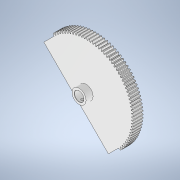
# Autodesk Inventor part: Spur Gear2
Saved by Autodesk Inventor 2020 (Build 240168000, 168)
## iProperties
CustomPartVersion: 1
Created: 2020-05-17
Part Number: Spur Gear2
Material: Acetal Resin, White
Document SubType Name: Modeling
Designer: Hesekiel
Categories: <?xml version="1.0" encoding="UTF-16"?> <MemberInstance><Categories><FamilyTemplate><FamilyTemplateParameter ValueType="xs:double" Id="1" ObjectReferenceKey="da_z" ObjectType="kUserParameterObject"/><FamilyTemplateParameter ValueType="xs:double" Id="2" ObjectReferenceKey="da_b" ObjectType="kUserParameterObject"/><FamilyTemplateParameter ValueType="xs:double" Id="3" ObjectReferenceKey="da_beta" ObjectType="kUserParameterObject"/><FamilyTemplateParameter ValueType="xs:double" Id="4" ObjectReferenceKey="da_da" ObjectType="kUserParameterObject"/><FamilyTemplateParameter ValueType="xs:double" Id="5" ObjectReferenceKey="da_aw" ObjectType="kUserParameterObject"/><FamilyTemplateParameter ValueType="xs:string" Id="6" ObjectReferenceKey="EAIAABAAAACIAQAAAAAAAIAAAAAAAAAA" ObjectType="83910656" SubObjectId="SurfaceGeometry"/></FamilyTemplate><ParamToTemplateMap><ParamToTemplate CategoryParameter="//CategoryParameter[@InternalName='046C89C9-8512-4d59-83FE-43B91F4F132A']" TemplateParameter="1"/><ParamToTemplate CategoryParameter="//CategoryParameter[@InternalName='2552DF32-E462-4b46-AEBF-C6C7768E72AC']" TemplateParameter="2"/><ParamToTemplate CategoryParameter="//CategoryParameter[@InternalName='C9EE641D-15FC-4fae-A226-E94C4372FDD7']" TemplateParameter="3"/><ParamToTemplate><ParamToTemplate CategoryParameter="//CategoryParameter[@InternalName='00B6519A-459B-49c7-AD84-2E56D39A5744']" ConstantValue="0.000000"/></ParamToTemplate><ParamToTemplate><ParamToTemplate CategoryParameter="//CategoryParameter[@InternalName='04B31F0E-C7A6-4894-AA32-9629BEFACF47']" ConstantValue="1.000000"/></ParamToTemplate><ParamToTemplate><ParamToTemplate CategoryParameter="//CategoryParameter[@InternalName='43CBEC2E-7847-49e7-A936-2F7889FCB2D9']" ConstantValue="0.250000"/></ParamToTemplate><ParamToTemplate><ParamToTemplate CategoryParameter="//CategoryParameter[@InternalName='B1EFC894-105D-4ebd-86BF-FA20ED196853']" ConstantValue="0.350000"/></ParamToTemplate><ParamToTemplate><ParamToTemplate CategoryParameter="//CategoryParameter[@InternalName='51175063-3D10-4879-93E8-6246FE8B403D']" ConstantValue="2060000000.000000"/></ParamToTemplate><ParamToTemplate><ParamToTemplate CategoryParameter="//CategoryParameter[@InternalName='A3A52E27-4454-46a9-B0BD-C932399B70AF']" ConstantValue="0.300000"/></ParamToTemplate><ParamToTemplate><ParamToTemplate CategoryParameter="//CategoryParameter[@InternalName='91B76062-C214-41d9-B1B9-14D2AB99603D']" ConstantValue="0.200000"/></ParamToTemplate><ParamToTemplate><ParamToTemplate CategoryParameter="//CategoryParameter[@InternalName='374E806E-8B8A-4dda-A9AA-1039D6500AD2']" ConstantValue="5.000000"/></ParamToTemplate><ParamToTemplate><ParamToTemplate CategoryParameter="//CategoryParameter[@InternalName='2D373A89-B862-43d6-8D0B-0CBF12AB9F6C']" ConstantValue="0.349066"/></ParamToTemplate><ParamToTemplate CategoryParameter="//CategoryParameter[@InternalName='37777632-D6A2-4fac-9D53-DB8ACD95C989']" TemplateParameter="4"/><ParamToTemplate CategoryParameter="//CategoryParameter[@InternalName='FD1017F1-B727-4f7e-9707-0F86F1FF9423']" TemplateParameter="5"/><ParamToTemplate><ParamToTemplate CategoryParameter="//CategoryParameter[@InternalName='9E1B4470-B2D3-4ff1-B813-535BB4CDF51A']" ConstantValue="3520000.000000"/></ParamToTemplate><ParamToTemplate><ParamToTemplate CategoryParameter="//CategoryParameter[@InternalName='F8452263-BFF6-458c-9FB1-07C4B99E95CD']" ConstantValue="11400000.000000"/></ParamToTemplate><ParamToTemplate><ParamToTemplate CategoryParameter="//CategoryParameter[@InternalName='3E3BB259-FD49-497f-8171-6EBC954A3479']" ConstantValue="2.000000"/></ParamToTemplate><ParamToTemplate CategoryParameter="//CategoryParameter[@InternalName='27C3BAF2-7550-4e4b-AE2C-0DB134B7D9B7']" TemplateParameter="6"/></ParamToTemplateMap><Category DisplayName="Gear" InternalName="DC85795E-93AB-48d5-8EEE-5A27447B64BD" Mnemonic="Gear"><CategoryParameter DisplayName="z" InternalName="046C89C9-8512-4d59-83FE-43B91F4F132A" Mnemonic="z"/><CategoryParameter DisplayName="b" InternalName="2552DF32-E462-4b46-AEBF-C6C7768E72AC" Mnemonic="b"/><CategoryParameter DisplayName="||b|" InternalName="C9EE641D-15FC-4fae-A226-E94C4372FDD7" Mnemonic="beta"/><CategoryParameter DisplayName="x" InternalName="00B6519A-459B-49c7-AD84-2E56D39A5744" Mnemonic="x"/><CategoryParameter DisplayName="a*" InternalName="04B31F0E-C7A6-4894-AA32-9629BEFACF47" Mnemonic="a"/><CategoryParameter DisplayName="c*" InternalName="43CBEC2E-7847-49e7-A936-2F7889FCB2D9" Mnemonic="c"/><CategoryParameter DisplayName="r|.f|*" InternalName="B1EFC894-105D-4ebd-86BF-FA20ED196853" Mnemonic="rf"/><CategoryParameter DisplayName="E" InternalName="51175063-3D10-4879-93E8-6246FE8B403D" Mnemonic="E"/><CategoryParameter DisplayName="||m|" InternalName="A3A52E27-4454-46a9-B0BD-C932399B70AF" Mnemonic="mi"/><Category DisplayName="SpurGear" InternalName="26C5A22E-A91E-4dfd-A3B3-23CCAFAE1764" Mnemonic="SpurGear"><CategoryParameter DisplayName="m" InternalName="91B76062-C214-41d9-B1B9-14D2AB99603D" Mnemonic="m"/><CategoryParameter DisplayName="P" InternalName="374E806E-8B8A-4dda-A9AA-1039D6500AD2" Mnemonic="PP"/><CategoryParameter DisplayName="||a|" InternalName="2D373A89-B862-43d6-8D0B-0CBF12AB9F6C" Mnemonic="alpha"/><CategoryParameter DisplayName="d|.a|" InternalName="37777632-D6A2-4fac-9D53-DB8ACD95C989" Mnemonic="da"/><CategoryParameter DisplayName="a|.w|" InternalName="FD1017F1-B727-4f7e-9707-0F86F1FF9423" Mnemonic="aw"/><CategoryParameter DisplayName="||s||.Flim|" InternalName="9E1B4470-B2D3-4ff1-B813-535BB4CDF51A" Mnemonic="sFlim"/><CategoryParameter DisplayName="||s||.Hlim|" InternalName="F8452263-BFF6-458c-9FB1-07C4B99E95CD" Mnemonic="sHlim"/><CategoryParameter DisplayName="type" InternalName="3E3BB259-FD49-497f-8171-6EBC954A3479" Mnemonic="type"/><CategoryParameter DisplayName="PitchDiameter" InternalName="27C3BAF2-7550-4e4b-AE2C-0DB134B7D9B7" Mnemonic="IDS_PITCHDIAM"/></Category></Category></Categories></MemberInstance>
Density: 1.425 g/cm^3
Appearance: Smooth - White
Mass: 609.034 g
Surface Area: 653.622 cm^2
Volume: 427.392 cm^3
Author: Hesekiel
Autodesk Inventor part; units mm, degrees
(part 1 of 3)
ref_plane "YZ Plane" through (0, 0, 0) normal (1, 0, 0) x (0, 1, 0)
ref_plane "XZ Plane" through (0, 0, 0) normal (0, 1, 0) x (-1, 0, 0)
ref_plane "XY Plane" through (0, 0, 0) normal (0, 0, 1) x (1, 0, 0)
sketch "Sketch1" plane through (0, 0, 0) normal (0, 0, 1) x (1, 0, 0)
  circle A0 centre (0, 0) radius 102
  dimension "d0" = 204
  constraints: 1 centre point
  measures "d0" diameter of A0
extrude "Extrusion1" add sketch "Sketch1" along normal blind 20
ref_plane "Work Plane2" through (0, 0, 10) normal (0, 0, 1) x (1, 0, 0)
sketch "Sketch2" plane through (0, 0, 0) normal (0, 0, -1) x (-1, 0, 0)
  circle A0 centre (0, 0) radius 102 projected
  circle A1 centre (0, 0) radius 100
  dimension "d3" = 200
  constraints: 1 centre point, 1 coincident
  measures "d3" diameter of A1
surface extrude "Pitch Diameter" sketch "Sketch2" against normal through all shown no curves A1
ref_plane "Work Plane8" through (0, 0, 0) normal (0.9995066, 0.0314108, 0) x (0, 0, 1)
ref_plane "Work Plane9" through (0, 0, 0) normal (1, 0, 0) x (0, 1, 0)
spur gear teeth "Spur Gear" teeth 100 pitch diameter 200 tip diameter 204 root diameter 195 face width 20 start plane through (0, 0, 0) normal (0, 0, -1) x (-1, 0, 0)
sketch "Sketch3" plane through (0, 0, 20) normal (0, 0, 1) x (1, 0, 0)
  line L0 (0, 0) -> (-68.9429, 68.9429)
  arc A0 (-68.3993, 69.4823) -> (-69.4823, 68.3993) centre (0, 0) ccw projected
  line L1 (0, 0) -> (97.5, 0) construction
  line L2 (0, 0) -> (68.9429, -68.9429)
  arc A1 (68.3993, -69.4823) -> (69.4823, -68.3993) centre (0, 0) ccw projected
  line L3 (0, 0) -> (97.5, 0) construction
  arc A2 (-7.204, 101.7453) -> (-8.4129, 97.1364) centre (19.356, 92.3153) ccw projected
  arc A3 (-8.4129, 97.1364) -> (-9.9376, 96.9922) centre (0, 0) ccw projected
  arc A4 (-9.9376, 96.9922) -> (-11.9888, 101.293) centre (-36.3113, 87.0532) ccw projected
  arc A5 (-11.9888, 101.293) -> (-13.5784, 101.0922) centre (0, 0) ccw projected
  arc A6 (-13.5784, 101.0922) -> (-14.4956, 96.4164) centre (13.5213, 93.3485) ccw projected
  arc A7 (-14.4956, 96.4164) -> (-16.0082, 96.1769) centre (0, 0) ccw projected
  arc A8 (-16.0082, 96.1769) -> (-18.3254, 100.3403) centre (-41.7058, 84.6014) ccw projected
  arc A9 (-18.3254, 100.3403) -> (-19.8992, 100.0401) centre (0, 0) ccw projected
  arc A10 (-19.8992, 100.0401) -> (-20.521, 95.316) centre (7.6332, 94.0133) ccw projected
  arc A11 (-20.521, 95.316) -> (-22.0156, 94.9819) centre (0, 0) ccw projected
  arc A12 (-22.0156, 94.9819) -> (-24.5897, 98.9917) centre (-46.9356, 81.8157) ccw projected
  arc A13 (-24.5897, 98.9917) -> (-26.1415, 98.5932) centre (0, 0) ccw projected
  arc A14 (-26.1415, 98.5932) -> (-26.4654, 93.8394) centre (1.715, 94.3071) ccw projected
  arc A15 (-26.4654, 93.8394) -> (-27.9361, 93.4121) centre (0, 0) ccw projected
  arc A16 (-27.9361, 93.4121) -> (-30.7569, 97.2523) centre (-51.9803, 78.7072) ccw projected
  arc A17 (-30.7569, 97.2523) -> (-32.2807, 96.7572) centre (0, 0) ccw projected
  arc A18 (-32.2807, 96.7572) -> (-32.3054, 91.9924) centre (-4.21, 94.2287) ccw projected
  arc A19 (-32.3054, 91.9924) -> (-33.7464, 91.4737) centre (0, 0) ccw projected
  arc A20 (-33.7464, 91.4737) -> (-36.8027, 95.1292) centre (-56.8198, 75.288) ccw projected
  arc A21 (-36.8027, 95.1292) -> (-38.2924, 94.5394) centre (0, 0) ccw projected
  arc A22 (-38.2924, 94.5394) -> (-38.0179, 89.7824) centre (-10.1184, 93.7784) ccw projected
  arc A23 (-38.0179, 89.7824) -> (-39.4235, 89.1742) centre (0, 0) ccw projected
  arc A24 (-39.4235, 89.1742) -> (-42.7033, 92.6306) centre (-61.435, 71.5717) ccw projected
  arc A25 (-42.7033, 92.6306) -> (-44.153, 91.9484) centre (0, 0) ccw projected
  arc A26 (-44.153, 91.9484) -> (-43.5804, 87.2181) centre (-15.9868, 92.958) ccw projected
  arc A27 (-43.5804, 87.2181) -> (-44.945, 86.5228) centre (0, 0) ccw projected
  arc A28 (-44.945, 86.5228) -> (-48.4354, 89.7665) centre (-65.8078, 67.5729) ccw projected
  arc A29 (-48.4354, 89.7665) -> (-49.8394, 88.9946) centre (0, 0) ccw projected
  arc A30 (-49.8394, 88.9946) -> (-48.9709, 84.3096) centre (-21.7921, 91.7708) ccw projected
  arc A31 (-48.9709, 84.3096) -> (-50.2891, 83.53) centre (0, 0) ccw projected
  arc A32 (-50.2891, 83.53) -> (-53.9763, 86.548) centre (-69.9209, 63.3075) ccw projected
  arc A33 (-53.9763, 86.548) -> (-55.329, 85.6895) centre (0, 0) ccw projected
  arc A34 (-55.329, 85.6895) -> (-54.1681, 81.0683) centre (-27.5115, 90.2213) ccw projected
  arc A35 (-54.1681, 81.0683) -> (-55.4348, 80.2075) centre (0, 0) ccw projected
  arc A36 (-55.4348, 80.2075) -> (-59.3041, 82.9881) centre (-73.758, 58.7922) ccw projected
  arc A37 (-59.3041, 82.9881) -> (-60.6003, 82.0463) centre (0, 0) ccw projected
  arc A38 (-60.6003, 82.0463) -> (-59.1515, 77.5071) centre (-33.1222, 88.3159) ccw projected
  arc A39 (-59.1515, 77.5071) -> (-60.3617, 76.5684) centre (0, 0) ccw projected
  arc A40 (-60.3617, 76.5684) -> (-64.398, 79.1006) centre (-77.3041, 54.0449) ccw projected
  arc A41 (-64.398, 79.1006) -> (-65.6325, 78.0793) centre (0, 0) ccw projected
  arc A42 (-65.6325, 78.0793) -> (-63.9015, 73.64) centre (-38.6023, 86.0618) ccw projected
  arc A43 (-63.9015, 73.64) -> (-65.0503, 72.6272) centre (0, 0) ccw projected
  arc A44 (-65.0503, 72.6272) -> (-69.2377, 74.9009) centre (-80.5451, 49.0843) ccw projected
  arc A45 (-69.2377, 74.9009) -> (-70.4056, 73.8041) centre (0, 0) ccw projected
  arc A46 (-70.4056, 73.8041) -> (-68.3993, 69.4823) centre (-43.9299, 83.4681) ccw projected
  arc A47 (-68.3993, 69.4823) -> (-69.4823, 68.3993) centre (0, 0) ccw projected
  arc A48 (-69.4823, 68.3993) -> (-73.8041, 70.4056) centre (-83.4681, 43.9299) ccw projected
  arc A49 (-73.8041, 70.4056) -> (-74.9009, 69.2377) centre (0, 0) ccw projected
  arc A50 (-74.9009, 69.2377) -> (-72.6272, 65.0503) centre (-49.0843, 80.5451) ccw projected
  arc A51 (-72.6272, 65.0503) -> (-73.64, 63.9015) centre (0, 0) ccw projected
  arc A52 (-73.64, 63.9015) -> (-78.0793, 65.6325) centre (-86.0618, 38.6023) ccw projected
  arc A53 (-78.0793, 65.6325) -> (-79.1006, 64.398) centre (0, 0) ccw projected
  arc A54 (-79.1006, 64.398) -> (-76.5684, 60.3617) centre (-54.0449, 77.3041) ccw projected
  arc A55 (-76.5684, 60.3617) -> (-77.5071, 59.1515) centre (0, 0) ccw projected
  arc A56 (-77.5071, 59.1515) -> (-82.0463, 60.6003) centre (-88.3159, 33.1222) ccw projected
  arc A57 (-82.0463, 60.6003) -> (-82.9881, 59.3041) centre (0, 0) ccw projected
  arc A58 (-82.9881, 59.3041) -> (-80.2075, 55.4348) centre (-58.7922, 73.758) ccw projected
  arc A59 (-80.2075, 55.4348) -> (-81.0683, 54.1681) centre (0, 0) ccw projected
  arc A60 (-81.0683, 54.1681) -> (-85.6895, 55.329) centre (-90.2213, 27.5115) ccw projected
  arc A61 (-85.6895, 55.329) -> (-86.548, 53.9763) centre (0, 0) ccw projected
  arc A62 (-86.548, 53.9763) -> (-83.53, 50.2891) centre (-63.3075, 69.9209) ccw projected
  arc A63 (-83.53, 50.2891) -> (-84.3096, 48.9709) centre (0, 0) ccw projected
  arc A64 (-84.3096, 48.9709) -> (-88.9946, 49.8394) centre (-91.7708, 21.7921) ccw projected
  arc A65 (-88.9946, 49.8394) -> (-89.7665, 48.4354) centre (0, 0) ccw projected
  arc A66 (-89.7665, 48.4354) -> (-86.5228, 44.945) centre (-67.5729, 65.8078) ccw projected
  arc A67 (-86.5228, 44.945) -> (-87.2181, 43.5804) centre (0, 0) ccw projected
  arc A68 (-87.2181, 43.5804) -> (-91.9484, 44.153) centre (-92.958, 15.9868) ccw projected
  arc A69 (-91.9484, 44.153) -> (-92.6306, 42.7033) centre (0, 0) ccw projected
  arc A70 (-92.6306, 42.7033) -> (-89.1742, 39.4235) centre (-71.5717, 61.435) ccw projected
  arc A71 (-89.1742, 39.4235) -> (-89.7824, 38.0179) centre (0, 0) ccw projected
  arc A72 (-89.7824, 38.0179) -> (-94.5394, 38.2924) centre (-93.7784, 10.1184) ccw projected
  arc A73 (-94.5394, 38.2924) -> (-95.1292, 36.8027) centre (0, 0) ccw projected
  arc A74 (-95.1292, 36.8027) -> (-91.4737, 33.7464) centre (-75.288, 56.8198) ccw projected
  arc A75 (-91.4737, 33.7464) -> (-91.9924, 32.3054) centre (0, 0) ccw projected
  arc A76 (-91.9924, 32.3054) -> (-96.7572, 32.2807) centre (-94.2287, 4.21) ccw projected
  arc A77 (-96.7572, 32.2807) -> (-97.2523, 30.7569) centre (0, 0) ccw projected
  arc A78 (-97.2523, 30.7569) -> (-93.4121, 27.9361) centre (-78.7072, 51.9803) ccw projected
  arc A79 (-93.4121, 27.9361) -> (-93.8394, 26.4654) centre (0, 0) ccw projected
  arc A80 (-93.8394, 26.4654) -> (-98.5932, 26.1415) centre (-94.3071, -1.715) ccw projected
  arc A81 (-98.5932, 26.1415) -> (-98.9917, 24.5897) centre (0, 0) ccw projected
  arc A82 (-98.9917, 24.5897) -> (-94.9819, 22.0156) centre (-81.8157, 46.9356) ccw projected
  arc A83 (-94.9819, 22.0156) -> (-95.316, 20.521) centre (0, 0) ccw projected
  arc A84 (-95.316, 20.521) -> (-100.0401, 19.8992) centre (-94.0133, -7.6332) ccw projected
  arc A85 (-100.0401, 19.8992) -> (-100.3403, 18.3254) centre (0, 0) ccw projected
  arc A86 (-100.3403, 18.3254) -> (-96.1769, 16.0082) centre (-84.6014, 41.7058) ccw projected
  arc A87 (-96.1769, 16.0082) -> (-96.4164, 14.4956) centre (0, 0) ccw projected
  arc A88 (-96.4164, 14.4956) -> (-101.0922, 13.5784) centre (-93.3485, -13.5213) ccw projected
  arc A89 (-101.0922, 13.5784) -> (-101.293, 11.9888) centre (0, 0) ccw projected
  arc A90 (-101.293, 11.9888) -> (-96.9922, 9.9376) centre (-87.0532, 36.3113) ccw projected
  arc A91 (-96.9922, 9.9376) -> (-97.1364, 8.4129) centre (0, 0) ccw projected
  arc A92 (-97.1364, 8.4129) -> (-101.7453, 7.204) centre (-92.3153, -19.356) ccw projected
  arc A93 (-101.7453, 7.204) -> (-101.8459, 5.6049) centre (0, 0) ccw projected
  arc A94 (-101.8459, 5.6049) -> (-97.4248, 3.8278) centre (-89.1614, 30.7735) ccw projected
  arc A95 (-97.4248, 3.8278) -> (-97.4729, 2.2971) centre (0, 0) ccw projected
  arc A96 (-97.4729, 2.2971) -> (-101.9969, 0.8011) centre (-90.9178, -25.1143) ccw projected
  arc A97 (-101.9969, 0.8011) -> (-101.9969, -0.8011) centre (0, 0) ccw projected
  arc A98 (-101.9969, -0.8011) -> (-97.4729, -2.2971) centre (-90.9178, 25.1143) ccw projected
  arc A99 (-97.4729, -2.2971) -> (-97.4248, -3.8278) centre (0, 0) ccw projected
  arc A100 (-97.4248, -3.8278) -> (-101.8459, -5.6049) centre (-89.1614, -30.7735) ccw projected
  arc A101 (-101.8459, -5.6049) -> (-101.7453, -7.204) centre (0, 0) ccw projected
  arc A102 (-101.7453, -7.204) -> (-97.1364, -8.4129) centre (-92.3153, 19.356) ccw projected
  arc A103 (-97.1364, -8.4129) -> (-96.9922, -9.9376) centre (0, 0) ccw projected
  arc A104 (-96.9922, -9.9376) -> (-101.293, -11.9888) centre (-87.0532, -36.3113) ccw projected
  arc A105 (-101.293, -11.9888) -> (-101.0922, -13.5784) centre (0, 0) ccw projected
  arc A106 (-101.0922, -13.5784) -> (-96.4164, -14.4956) centre (-93.3485, 13.5213) ccw projected
  arc A107 (-96.4164, -14.4956) -> (-96.1769, -16.0082) centre (0, 0) ccw projected
  arc A108 (-96.1769, -16.0082) -> (-100.3403, -18.3254) centre (-84.6014, -41.7058) ccw projected
  arc A109 (-100.3403, -18.3254) -> (-100.0401, -19.8992) centre (0, 0) ccw projected
  arc A110 (-100.0401, -19.8992) -> (-95.316, -20.521) centre (-94.0133, 7.6332) ccw projected
  arc A111 (-95.316, -20.521) -> (-94.9819, -22.0156) centre (0, 0) ccw projected
  arc A112 (-94.9819, -22.0156) -> (-98.9917, -24.5897) centre (-81.8157, -46.9356) ccw projected
  arc A113 (-98.9917, -24.5897) -> (-98.5932, -26.1415) centre (0, 0) ccw projected
  arc A114 (-98.5932, -26.1415) -> (-93.8394, -26.4654) centre (-94.3071, 1.715) ccw projected
  arc A115 (-93.8394, -26.4654) -> (-93.4121, -27.9361) centre (0, 0) ccw projected
  arc A116 (-93.4121, -27.9361) -> (-97.2523, -30.7569) centre (-78.7072, -51.9803) ccw projected
  arc A117 (-97.2523, -30.7569) -> (-96.7572, -32.2807) centre (0, 0) ccw projected
  arc A118 (-96.7572, -32.2807) -> (-91.9924, -32.3054) centre (-94.2287, -4.21) ccw projected
  arc A119 (-91.9924, -32.3054) -> (-91.4737, -33.7464) centre (0, 0) ccw projected
  arc A120 (-91.4737, -33.7464) -> (-95.1292, -36.8027) centre (-75.288, -56.8198) ccw projected
  arc A121 (-95.1292, -36.8027) -> (-94.5394, -38.2924) centre (0, 0) ccw projected
  arc A122 (-94.5394, -38.2924) -> (-89.7824, -38.0179) centre (-93.7784, -10.1184) ccw projected
  arc A123 (-89.7824, -38.0179) -> (-89.1742, -39.4235) centre (0, 0) ccw projected
  arc A124 (-89.1742, -39.4235) -> (-92.6306, -42.7033) centre (-71.5717, -61.435) ccw projected
  arc A125 (-92.6306, -42.7033) -> (-91.9484, -44.153) centre (0, 0) ccw projected
  arc A126 (-91.9484, -44.153) -> (-87.2181, -43.5804) centre (-92.958, -15.9868) ccw projected
  arc A127 (-87.2181, -43.5804) -> (-86.5228, -44.945) centre (0, 0) ccw projected
  arc A128 (-86.5228, -44.945) -> (-89.7665, -48.4354) centre (-67.5729, -65.8078) ccw projected
  arc A129 (-89.7665, -48.4354) -> (-88.9946, -49.8394) centre (0, 0) ccw projected
  arc A130 (-88.9946, -49.8394) -> (-84.3096, -48.9709) centre (-91.7708, -21.7921) ccw projected
  arc A131 (-84.3096, -48.9709) -> (-83.53, -50.2891) centre (0, 0) ccw projected
  arc A132 (-83.53, -50.2891) -> (-86.548, -53.9763) centre (-63.3075, -69.9209) ccw projected
  arc A133 (-86.548, -53.9763) -> (-85.6895, -55.329) centre (0, 0) ccw projected
  arc A134 (-85.6895, -55.329) -> (-81.0683, -54.1681) centre (-90.2213, -27.5115) ccw projected
  arc A135 (-81.0683, -54.1681) -> (-80.2075, -55.4348) centre (0, 0) ccw projected
  arc A136 (-80.2075, -55.4348) -> (-82.9881, -59.3041) centre (-58.7922, -73.758) ccw projected
  arc A137 (-82.9881, -59.3041) -> (-82.0463, -60.6003) centre (0, 0) ccw projected
  arc A138 (-82.0463, -60.6003) -> (-77.5071, -59.1515) centre (-88.3159, -33.1222) ccw projected
  arc A139 (-77.5071, -59.1515) -> (-76.5684, -60.3617) centre (0, 0) ccw projected
  arc A140 (-76.5684, -60.3617) -> (-79.1006, -64.398) centre (-54.0449, -77.3041) ccw projected
  arc A141 (-79.1006, -64.398) -> (-78.0793, -65.6325) centre (0, 0) ccw projected
  arc A142 (-78.0793, -65.6325) -> (-73.64, -63.9015) centre (-86.0618, -38.6023) ccw projected
  arc A143 (-73.64, -63.9015) -> (-72.6272, -65.0503) centre (0, 0) ccw projected
  arc A144 (-72.6272, -65.0503) -> (-74.9009, -69.2377) centre (-49.0843, -80.5451) ccw projected
  arc A145 (-74.9009, -69.2377) -> (-73.8041, -70.4056) centre (0, 0) ccw projected
  arc A146 (-73.8041, -70.4056) -> (-69.4823, -68.3993) centre (-83.4681, -43.9299) ccw projected
  arc A147 (-69.4823, -68.3993) -> (-68.3993, -69.4823) centre (0, 0) ccw projected
  arc A148 (-68.3993, -69.4823) -> (-70.4056, -73.8041) centre (-43.9299, -83.4681) ccw projected
  arc A149 (-70.4056, -73.8041) -> (-69.2377, -74.9009) centre (0, 0) ccw projected
  arc A150 (-69.2377, -74.9009) -> (-65.0503, -72.6272) centre (-80.5451, -49.0843) ccw projected
  arc A151 (-65.0503, -72.6272) -> (-63.9015, -73.64) centre (0, 0) ccw projected
  arc A152 (-63.9015, -73.64) -> (-65.6325, -78.0793) centre (-38.6023, -86.0618) ccw projected
  arc A153 (-65.6325, -78.0793) -> (-64.398, -79.1006) centre (0, 0) ccw projected
  arc A154 (-64.398, -79.1006) -> (-60.3617, -76.5684) centre (-77.3041, -54.0449) ccw projected
  arc A155 (-60.3617, -76.5684) -> (-59.1515, -77.5071) centre (0, 0) ccw projected
  arc A156 (-59.1515, -77.5071) -> (-60.6003, -82.0463) centre (-33.1222, -88.3159) ccw projected
  arc A157 (-60.6003, -82.0463) -> (-59.3041, -82.9881) centre (0, 0) ccw projected
  arc A158 (-59.3041, -82.9881) -> (-55.4348, -80.2075) centre (-73.758, -58.7922) ccw projected
  arc A159 (-55.4348, -80.2075) -> (-54.1681, -81.0683) centre (0, 0) ccw projected
  arc A160 (-54.1681, -81.0683) -> (-55.329, -85.6895) centre (-27.5115, -90.2213) ccw projected
  arc A161 (-55.329, -85.6895) -> (-53.9763, -86.548) centre (0, 0) ccw projected
  arc A162 (-53.9763, -86.548) -> (-50.2891, -83.53) centre (-69.9209, -63.3075) ccw projected
  arc A163 (-50.2891, -83.53) -> (-48.9709, -84.3096) centre (0, 0) ccw projected
  arc A164 (-48.9709, -84.3096) -> (-49.8394, -88.9946) centre (-21.7921, -91.7708) ccw projected
  arc A165 (-49.8394, -88.9946) -> (-48.4354, -89.7665) centre (0, 0) ccw projected
  arc A166 (-48.4354, -89.7665) -> (-44.945, -86.5228) centre (-65.8078, -67.5729) ccw projected
  arc A167 (-44.945, -86.5228) -> (-43.5804, -87.2181) centre (0, 0) ccw projected
  arc A168 (-43.5804, -87.2181) -> (-44.153, -91.9484) centre (-15.9868, -92.958) ccw projected
  arc A169 (-44.153, -91.9484) -> (-42.7033, -92.6306) centre (0, 0) ccw projected
  arc A170 (-42.7033, -92.6306) -> (-39.4235, -89.1742) centre (-61.435, -71.5717) ccw projected
  arc A171 (-39.4235, -89.1742) -> (-38.0179, -89.7824) centre (0, 0) ccw projected
  arc A172 (-38.0179, -89.7824) -> (-38.2924, -94.5394) centre (-10.1184, -93.7784) ccw projected
  arc A173 (-38.2924, -94.5394) -> (-36.8027, -95.1292) centre (0, 0) ccw projected
  arc A174 (-36.8027, -95.1292) -> (-33.7464, -91.4737) centre (-56.8198, -75.288) ccw projected
  arc A175 (-33.7464, -91.4737) -> (-32.3054, -91.9924) centre (0, 0) ccw projected
  arc A176 (-32.3054, -91.9924) -> (-32.2807, -96.7572) centre (-4.21, -94.2287) ccw projected
  arc A177 (-32.2807, -96.7572) -> (-30.7569, -97.2523) centre (0, 0) ccw projected
  arc A178 (-30.7569, -97.2523) -> (-27.9361, -93.4121) centre (-51.9803, -78.7072) ccw projected
  arc A179 (-27.9361, -93.4121) -> (-26.4654, -93.8394) centre (0, 0) ccw projected
  arc A180 (-26.4654, -93.8394) -> (-26.1415, -98.5932) centre (1.715, -94.3071) ccw projected
  arc A181 (-26.1415, -98.5932) -> (-24.5897, -98.9917) centre (0, 0) ccw projected
  arc A182 (-24.5897, -98.9917) -> (-22.0156, -94.9819) centre (-46.9356, -81.8157) ccw projected
  arc A183 (-22.0156, -94.9819) -> (-20.521, -95.316) centre (0, 0) ccw projected
  arc A184 (-20.521, -95.316) -> (-19.8992, -100.0401) centre (7.6332, -94.0133) ccw projected
  arc A185 (-19.8992, -100.0401) -> (-18.3254, -100.3403) centre (0, 0) ccw projected
  arc A186 (-18.3254, -100.3403) -> (-16.0082, -96.1769) centre (-41.7058, -84.6014) ccw projected
  arc A187 (-16.0082, -96.1769) -> (-14.4956, -96.4164) centre (0, 0) ccw projected
  arc A188 (-14.4956, -96.4164) -> (-13.5784, -101.0922) centre (13.5213, -93.3485) ccw projected
  arc A189 (-13.5784, -101.0922) -> (-11.9888, -101.293) centre (0, 0) ccw projected
  arc A190 (-11.9888, -101.293) -> (-9.9376, -96.9922) centre (-36.3113, -87.0532) ccw projected
  arc A191 (-9.9376, -96.9922) -> (-8.4129, -97.1364) centre (0, 0) ccw projected
  arc A192 (-8.4129, -97.1364) -> (-7.204, -101.7453) centre (19.356, -92.3153) ccw projected
  arc A193 (-7.204, -101.7453) -> (-5.6049, -101.8459) centre (0, 0) ccw projected
  arc A194 (-5.6049, -101.8459) -> (-3.8278, -97.4248) centre (-30.7735, -89.1614) ccw projected
  arc A195 (-3.8278, -97.4248) -> (-2.2971, -97.4729) centre (0, 0) ccw projected
  arc A196 (-2.2971, -97.4729) -> (-0.8011, -101.9969) centre (25.1143, -90.9178) ccw projected
  arc A197 (-0.8011, -101.9969) -> (0.8011, -101.9969) centre (0, 0) ccw projected
  arc A198 (0.8011, -101.9969) -> (2.2971, -97.4729) centre (-25.1143, -90.9178) ccw projected
  arc A199 (2.2971, -97.4729) -> (3.8278, -97.4248) centre (0, 0) ccw projected
  arc A200 (3.8278, -97.4248) -> (5.6049, -101.8459) centre (30.7735, -89.1614) ccw projected
  arc A201 (5.6049, -101.8459) -> (7.204, -101.7453) centre (0, 0) ccw projected
  arc A202 (7.204, -101.7453) -> (8.4129, -97.1364) centre (-19.356, -92.3153) ccw projected
  arc A203 (8.4129, -97.1364) -> (9.9376, -96.9922) centre (0, 0) ccw projected
  arc A204 (9.9376, -96.9922) -> (11.9888, -101.293) centre (36.3113, -87.0532) ccw projected
  arc A205 (11.9888, -101.293) -> (13.5784, -101.0922) centre (0, 0) ccw projected
  arc A206 (13.5784, -101.0922) -> (14.4956, -96.4164) centre (-13.5213, -93.3485) ccw projected
  arc A207 (14.4956, -96.4164) -> (16.0082, -96.1769) centre (0, 0) ccw projected
  arc A208 (16.0082, -96.1769) -> (18.3254, -100.3403) centre (41.7058, -84.6014) ccw projected
  arc A209 (18.3254, -100.3403) -> (19.8992, -100.0401) centre (0, 0) ccw projected
  arc A210 (19.8992, -100.0401) -> (20.521, -95.316) centre (-7.6332, -94.0133) ccw projected
  arc A211 (20.521, -95.316) -> (22.0156, -94.9819) centre (0, 0) ccw projected
  arc A212 (22.0156, -94.9819) -> (24.5897, -98.9917) centre (46.9356, -81.8157) ccw projected
  arc A213 (24.5897, -98.9917) -> (26.1415, -98.5932) centre (0, 0) ccw projected
  arc A214 (26.1415, -98.5932) -> (26.4654, -93.8394) centre (-1.715, -94.3071) ccw projected
  arc A215 (26.4654, -93.8394) -> (27.9361, -93.4121) centre (0, 0) ccw projected
  arc A216 (27.9361, -93.4121) -> (30.7569, -97.2523) centre (51.9803, -78.7072) ccw projected
  arc A217 (30.7569, -97.2523) -> (32.2807, -96.7572) centre (0, 0) ccw projected
  arc A218 (32.2807, -96.7572) -> (32.3054, -91.9924) centre (4.21, -94.2287) ccw projected
  arc A219 (32.3054, -91.9924) -> (33.7464, -91.4737) centre (0, 0) ccw projected
  arc A220 (33.7464, -91.4737) -> (36.8027, -95.1292) centre (56.8198, -75.288) ccw projected
  arc A221 (36.8027, -95.1292) -> (38.2924, -94.5394) centre (0, 0) ccw projected
  arc A222 (38.2924, -94.5394) -> (38.0179, -89.7824) centre (10.1184, -93.7784) ccw projected
  arc A223 (38.0179, -89.7824) -> (39.4235, -89.1742) centre (0, 0) ccw projected
  arc A224 (39.4235, -89.1742) -> (42.7033, -92.6306) centre (61.435, -71.5717) ccw projected
  arc A225 (42.7033, -92.6306) -> (44.153, -91.9484) centre (0, 0) ccw projected
  arc A226 (44.153, -91.9484) -> (43.5804, -87.2181) centre (15.9868, -92.958) ccw projected
  arc A227 (43.5804, -87.2181) -> (44.945, -86.5228) centre (0, 0) ccw projected
  arc A228 (44.945, -86.5228) -> (48.4354, -89.7665) centre (65.8078, -67.5729) ccw projected
  arc A229 (48.4354, -89.7665) -> (49.8394, -88.9946) centre (0, 0) ccw projected
  arc A230 (49.8394, -88.9946) -> (48.9709, -84.3096) centre (21.7921, -91.7708) ccw projected
  arc A231 (48.9709, -84.3096) -> (50.2891, -83.53) centre (0, 0) ccw projected
  arc A232 (50.2891, -83.53) -> (53.9763, -86.548) centre (69.9209, -63.3075) ccw projected
  arc A233 (53.9763, -86.548) -> (55.329, -85.6895) centre (0, 0) ccw projected
  arc A234 (55.329, -85.6895) -> (54.1681, -81.0683) centre (27.5115, -90.2213) ccw projected
  arc A235 (54.1681, -81.0683) -> (55.4348, -80.2075) centre (0, 0) ccw projected
  arc A236 (55.4348, -80.2075) -> (59.3041, -82.9881) centre (73.758, -58.7922) ccw projected
  arc A237 (59.3041, -82.9881) -> (60.6003, -82.0463) centre (0, 0) ccw projected
  arc A238 (60.6003, -82.0463) -> (59.1515, -77.5071) centre (33.1222, -88.3159) ccw projected
  arc A239 (59.1515, -77.5071) -> (60.3617, -76.5684) centre (0, 0) ccw projected
  arc A240 (60.3617, -76.5684) -> (64.398, -79.1006) centre (77.3041, -54.0449) ccw projected
  arc A241 (64.398, -79.1006) -> (65.6325, -78.0793) centre (0, 0) ccw projected
  arc A242 (65.6325, -78.0793) -> (63.9015, -73.64) centre (38.6023, -86.0618) ccw projected
  arc A243 (63.9015, -73.64) -> (65.0503, -72.6272) centre (0, 0) ccw projected
  arc A244 (65.0503, -72.6272) -> (69.2377, -74.9009) centre (80.5451, -49.0843) ccw projected
  arc A245 (69.2377, -74.9009) -> (70.4056, -73.8041) centre (0, 0) ccw projected
  arc A246 (70.4056, -73.8041) -> (68.3993, -69.4823) centre (43.9299, -83.4681) ccw projected
  arc A247 (68.3993, -69.4823) -> (69.4823, -68.3993) centre (0, 0) ccw projected
  arc A248 (69.4823, -68.3993) -> (73.8041, -70.4056) centre (83.4681, -43.9299) ccw projected
  arc A249 (73.8041, -70.4056) -> (74.9009, -69.2377) centre (0, 0) ccw projected
  arc A250 (74.9009, -69.2377) -> (72.6272, -65.0503) centre (49.0843, -80.5451) ccw projected
  arc A251 (72.6272, -65.0503) -> (73.64, -63.9015) centre (0, 0) ccw projected
  arc A252 (73.64, -63.9015) -> (78.0793, -65.6325) centre (86.0618, -38.6023) ccw projected
  arc A253 (78.0793, -65.6325) -> (79.1006, -64.398) centre (0, 0) ccw projected
  arc A254 (79.1006, -64.398) -> (76.5684, -60.3617) centre (54.0449, -77.3041) ccw projected
  arc A255 (76.5684, -60.3617) -> (77.5071, -59.1515) centre (0, 0) ccw projected
  arc A256 (77.5071, -59.1515) -> (82.0463, -60.6003) centre (88.3159, -33.1222) ccw projected
  arc A257 (82.0463, -60.6003) -> (82.9881, -59.3041) centre (0, 0) ccw projected
  arc A258 (82.9881, -59.3041) -> (80.2075, -55.4348) centre (58.7922, -73.758) ccw projected
  arc A259 (80.2075, -55.4348) -> (81.0683, -54.1681) centre (0, 0) ccw projected
  arc A260 (81.0683, -54.1681) -> (85.6895, -55.329) centre (90.2213, -27.5115) ccw projected
  arc A261 (85.6895, -55.329) -> (86.548, -53.9763) centre (0, 0) ccw projected
  arc A262 (86.548, -53.9763) -> (83.53, -50.2891) centre (63.3075, -69.9209) ccw projected
  arc A263 (83.53, -50.2891) -> (84.3096, -48.9709) centre (0, 0) ccw projected
  arc A264 (84.3096, -48.9709) -> (88.9946, -49.8394) centre (91.7708, -21.7921) ccw projected
  arc A265 (88.9946, -49.8394) -> (89.7665, -48.4354) centre (0, 0) ccw projected
  arc A266 (89.7665, -48.4354) -> (86.5228, -44.945) centre (67.5729, -65.8078) ccw projected
  arc A267 (86.5228, -44.945) -> (87.2181, -43.5804) centre (0, 0) ccw projected
  arc A268 (87.2181, -43.5804) -> (91.9484, -44.153) centre (92.958, -15.9868) ccw projected
  arc A269 (91.9484, -44.153) -> (92.6306, -42.7033) centre (0, 0) ccw projected
  arc A270 (92.6306, -42.7033) -> (89.1742, -39.4235) centre (71.5717, -61.435) ccw projected
  arc A271 (89.1742, -39.4235) -> (89.7824, -38.0179) centre (0, 0) ccw projected
  arc A272 (89.7824, -38.0179) -> (94.5394, -38.2924) centre (93.7784, -10.1184) ccw projected
  arc A273 (94.5394, -38.2924) -> (95.1292, -36.8027) centre (0, 0) ccw projected
  arc A274 (95.1292, -36.8027) -> (91.4737, -33.7464) centre (75.288, -56.8198) ccw projected
  arc A275 (91.4737, -33.7464) -> (91.9924, -32.3054) centre (0, 0) ccw projected
  arc A276 (91.9924, -32.3054) -> (96.7572, -32.2807) centre (94.2287, -4.21) ccw projected
  arc A277 (96.7572, -32.2807) -> (97.2523, -30.7569) centre (0, 0) ccw projected
  arc A278 (97.2523, -30.7569) -> (93.4121, -27.9361) centre (78.7072, -51.9803) ccw projected
  arc A279 (93.4121, -27.9361) -> (93.8394, -26.4654) centre (0, 0) ccw projected
  arc A280 (93.8394, -26.4654) -> (98.5932, -26.1415) centre (94.3071, 1.715) ccw projected
  arc A281 (98.5932, -26.1415) -> (98.9917, -24.5897) centre (0, 0) ccw projected
  arc A282 (98.9917, -24.5897) -> (94.9819, -22.0156) centre (81.8157, -46.9356) ccw projected
  arc A283 (94.9819, -22.0156) -> (95.316, -20.521) centre (0, 0) ccw projected
  arc A284 (95.316, -20.521) -> (100.0401, -19.8992) centre (94.0133, 7.6332) ccw projected
  arc A285 (100.0401, -19.8992) -> (100.3403, -18.3254) centre (0, 0) ccw projected
  arc A286 (100.3403, -18.3254) -> (96.1769, -16.0082) centre (84.6014, -41.7058) ccw projected
  arc A287 (96.1769, -16.0082) -> (96.4164, -14.4956) centre (0, 0) ccw projected
  arc A288 (96.4164, -14.4956) -> (101.0922, -13.5784) centre (93.3485, 13.5213) ccw projected
  arc A289 (101.0922, -13.5784) -> (101.293, -11.9888) centre (0, 0) ccw projected
  arc A290 (101.293, -11.9888) -> (96.9922, -9.9376) centre (87.0532, -36.3113) ccw projected
  arc A291 (96.9922, -9.9376) -> (97.1364, -8.4129) centre (0, 0) ccw projected
  arc A292 (97.1364, -8.4129) -> (101.7453, -7.204) centre (92.3153, 19.356) ccw projected
  arc A293 (101.7453, -7.204) -> (101.8459, -5.6049) centre (0, 0) ccw projected
  arc A294 (101.8459, -5.6049) -> (97.4248, -3.8278) centre (89.1614, -30.7735) ccw projected
  arc A295 (97.4248, -3.8278) -> (97.4729, -2.2971) centre (0, 0) ccw projected
  arc A296 (97.4729, -2.2971) -> (101.9969, -0.8011) centre (90.9178, 25.1143) ccw projected
  arc A297 (101.9969, -0.8011) -> (101.9969, 0.8011) centre (0, 0) ccw projected
  arc A298 (101.9969, 0.8011) -> (97.4729, 2.2971) centre (90.9178, -25.1143) ccw projected
  arc A299 (97.4729, 2.2971) -> (97.4248, 3.8278) centre (0, 0) ccw projected
  arc A300 (97.4248, 3.8278) -> (101.8459, 5.6049) centre (89.1614, 30.7735) ccw projected
  arc A301 (101.8459, 5.6049) -> (101.7453, 7.204) centre (0, 0) ccw projected
  arc A302 (101.7453, 7.204) -> (97.1364, 8.4129) centre (92.3153, -19.356) ccw projected
  arc A303 (97.1364, 8.4129) -> (96.9922, 9.9376) centre (0, 0) ccw projected
  arc A304 (96.9922, 9.9376) -> (101.293, 11.9888) centre (87.0532, 36.3113) ccw projected
  arc A305 (101.293, 11.9888) -> (101.0922, 13.5784) centre (0, 0) ccw projected
  arc A306 (101.0922, 13.5784) -> (96.4164, 14.4956) centre (93.3485, -13.5213) ccw projected
  arc A307 (96.4164, 14.4956) -> (96.1769, 16.0082) centre (0, 0) ccw projected
  arc A308 (96.1769, 16.0082) -> (100.3403, 18.3254) centre (84.6014, 41.7058) ccw projected
  arc A309 (100.3403, 18.3254) -> (100.0401, 19.8992) centre (0, 0) ccw projected
  arc A310 (100.0401, 19.8992) -> (95.316, 20.521) centre (94.0133, -7.6332) ccw projected
  arc A311 (95.316, 20.521) -> (94.9819, 22.0156) centre (0, 0) ccw projected
  arc A312 (94.9819, 22.0156) -> (98.9917, 24.5897) centre (81.8157, 46.9356) ccw projected
  arc A313 (98.9917, 24.5897) -> (98.5932, 26.1415) centre (0, 0) ccw projected
  arc A314 (98.5932, 26.1415) -> (93.8394, 26.4654) centre (94.3071, -1.715) ccw projected
  arc A315 (93.8394, 26.4654) -> (93.4121, 27.9361) centre (0, 0) ccw projected
  arc A316 (93.4121, 27.9361) -> (97.2523, 30.7569) centre (78.7072, 51.9803) ccw projected
  arc A317 (97.2523, 30.7569) -> (96.7572, 32.2807) centre (0, 0) ccw projected
  arc A318 (96.7572, 32.2807) -> (91.9924, 32.3054) centre (94.2287, 4.21) ccw projected
  arc A319 (91.9924, 32.3054) -> (91.4737, 33.7464) centre (0, 0) ccw projected
  arc A320 (91.4737, 33.7464) -> (95.1292, 36.8027) centre (75.288, 56.8198) ccw projected
  arc A321 (95.1292, 36.8027) -> (94.5394, 38.2924) centre (0, 0) ccw projected
  arc A322 (94.5394, 38.2924) -> (89.7824, 38.0179) centre (93.7784, 10.1184) ccw projected
  arc A323 (89.7824, 38.0179) -> (89.1742, 39.4235) centre (0, 0) ccw projected
  arc A324 (89.1742, 39.4235) -> (92.6306, 42.7033) centre (71.5717, 61.435) ccw projected
  arc A325 (92.6306, 42.7033) -> (91.9484, 44.153) centre (0, 0) ccw projected
  arc A326 (91.9484, 44.153) -> (87.2181, 43.5804) centre (92.958, 15.9868) ccw projected
  arc A327 (87.2181, 43.5804) -> (86.5228, 44.945) centre (0, 0) ccw projected
  arc A328 (86.5228, 44.945) -> (89.7665, 48.4354) centre (67.5729, 65.8078) ccw projected
  arc A329 (89.7665, 48.4354) -> (88.9946, 49.8394) centre (0, 0) ccw projected
  arc A330 (88.9946, 49.8394) -> (84.3096, 48.9709) centre (91.7708, 21.7921) ccw projected
  arc A331 (84.3096, 48.9709) -> (83.53, 50.2891) centre (0, 0) ccw projected
  arc A332 (83.53, 50.2891) -> (86.548, 53.9763) centre (63.3075, 69.9209) ccw projected
  arc A333 (86.548, 53.9763) -> (85.6895, 55.329) centre (0, 0) ccw projected
  arc A334 (85.6895, 55.329) -> (81.0683, 54.1681) centre (90.2213, 27.5115) ccw projected
  arc A335 (81.0683, 54.1681) -> (80.2075, 55.4348) centre (0, 0) ccw projected
  arc A336 (80.2075, 55.4348) -> (82.9881, 59.3041) centre (58.7922, 73.758) ccw projected
  arc A337 (82.9881, 59.3041) -> (82.0463, 60.6003) centre (0, 0) ccw projected
  arc A338 (82.0463, 60.6003) -> (77.5071, 59.1515) centre (88.3159, 33.1222) ccw projected
  arc A339 (77.5071, 59.1515) -> (76.5684, 60.3617) centre (0, 0) ccw projected
  arc A340 (76.5684, 60.3617) -> (79.1006, 64.398) centre (54.0449, 77.3041) ccw projected
  arc A341 (79.1006, 64.398) -> (78.0793, 65.6325) centre (0, 0) ccw projected
  arc A342 (78.0793, 65.6325) -> (73.64, 63.9015) centre (86.0618, 38.6023) ccw projected
  arc A343 (73.64, 63.9015) -> (72.6272, 65.0503) centre (0, 0) ccw projected
  arc A344 (72.6272, 65.0503) -> (74.9009, 69.2377) centre (49.0843, 80.5451) ccw projected
  arc A345 (74.9009, 69.2377) -> (73.8041, 70.4056) centre (0, 0) ccw projected
  arc A346 (73.8041, 70.4056) -> (69.4823, 68.3993) centre (83.4681, 43.9299) ccw projected
  arc A347 (69.4823, 68.3993) -> (68.3993, 69.4823) centre (0, 0) ccw projected
  arc A348 (68.3993, 69.4823) -> (70.4056, 73.8041) centre (43.9299, 83.4681) ccw projected
  arc A349 (70.4056, 73.8041) -> (69.2377, 74.9009) centre (0, 0) ccw projected
  arc A350 (69.2377, 74.9009) -> (65.0503, 72.6272) centre (80.5451, 49.0843) ccw projected
  arc A351 (65.0503, 72.6272) -> (63.9015, 73.64) centre (0, 0) ccw projected
  arc A352 (63.9015, 73.64) -> (65.6325, 78.0793) centre (38.6023, 86.0618) ccw projected
  arc A353 (65.6325, 78.0793) -> (64.398, 79.1006) centre (0, 0) ccw projected
  arc A354 (64.398, 79.1006) -> (60.3617, 76.5684) centre (77.3041, 54.0449) ccw projected
  arc A355 (60.3617, 76.5684) -> (59.1515, 77.5071) centre (0, 0) ccw projected
  arc A356 (59.1515, 77.5071) -> (60.6003, 82.0463) centre (33.1222, 88.3159) ccw projected
  arc A357 (60.6003, 82.0463) -> (59.3041, 82.9881) centre (0, 0) ccw projected
  arc A358 (59.3041, 82.9881) -> (55.4348, 80.2075) centre (73.758, 58.7922) ccw projected
  arc A359 (55.4348, 80.2075) -> (54.1681, 81.0683) centre (0, 0) ccw projected
  arc A360 (54.1681, 81.0683) -> (55.329, 85.6895) centre (27.5115, 90.2213) ccw projected
  arc A361 (55.329, 85.6895) -> (53.9763, 86.548) centre (0, 0) ccw projected
  arc A362 (53.9763, 86.548) -> (50.2891, 83.53) centre (69.9209, 63.3075) ccw projected
  arc A363 (50.2891, 83.53) -> (48.9709, 84.3096) centre (0, 0) ccw projected
  arc A364 (48.9709, 84.3096) -> (49.8394, 88.9946) centre (21.7921, 91.7708) ccw projected
  arc A365 (49.8394, 88.9946) -> (48.4354, 89.7665) centre (0, 0) ccw projected
  arc A366 (48.4354, 89.7665) -> (44.945, 86.5228) centre (65.8078, 67.5729) ccw projected
  arc A367 (44.945, 86.5228) -> (43.5804, 87.2181) centre (0, 0) ccw projected
  arc A368 (43.5804, 87.2181) -> (44.153, 91.9484) centre (15.9868, 92.958) ccw projected
  arc A369 (44.153, 91.9484) -> (42.7033, 92.6306) centre (0, 0) ccw projected
  arc A370 (42.7033, 92.6306) -> (39.4235, 89.1742) centre (61.435, 71.5717) ccw projected
  arc A371 (39.4235, 89.1742) -> (38.0179, 89.7824) centre (0, 0) ccw projected
  arc A372 (38.0179, 89.7824) -> (38.2924, 94.5394) centre (10.1184, 93.7784) ccw projected
  arc A373 (38.2924, 94.5394) -> (36.8027, 95.1292) centre (0, 0) ccw projected
  arc A374 (36.8027, 95.1292) -> (33.7464, 91.4737) centre (56.8198, 75.288) ccw projected
  arc A375 (33.7464, 91.4737) -> (32.3054, 91.9924) centre (0, 0) ccw projected
  arc A376 (32.3054, 91.9924) -> (32.2807, 96.7572) centre (4.21, 94.2287) ccw projected
  arc A377 (32.2807, 96.7572) -> (30.7569, 97.2523) centre (0, 0) ccw projected
  arc A378 (30.7569, 97.2523) -> (27.9361, 93.4121) centre (51.9803, 78.7072) ccw projected
  arc A379 (27.9361, 93.4121) -> (26.4654, 93.8394) centre (0, 0) ccw projected
  arc A380 (26.4654, 93.8394) -> (26.1415, 98.5932) centre (-1.715, 94.3071) ccw projected
  arc A381 (26.1415, 98.5932) -> (24.5897, 98.9917) centre (0, 0) ccw projected
  arc A382 (24.5897, 98.9917) -> (22.0156, 94.9819) centre (46.9356, 81.8157) ccw projected
  arc A383 (22.0156, 94.9819) -> (20.521, 95.316) centre (0, 0) ccw projected
  arc A384 (20.521, 95.316) -> (19.8992, 100.0401) centre (-7.6332, 94.0133) ccw projected
  arc A385 (19.8992, 100.0401) -> (18.3254, 100.3403) centre (0, 0) ccw projected
  arc A386 (18.3254, 100.3403) -> (16.0082, 96.1769) centre (41.7058, 84.6014) ccw projected
  arc A387 (16.0082, 96.1769) -> (14.4956, 96.4164) centre (0, 0) ccw projected
  arc A388 (14.4956, 96.4164) -> (13.5784, 101.0922) centre (-13.5213, 93.3485) ccw projected
  arc A389 (13.5784, 101.0922) -> (11.9888, 101.293) centre (0, 0) ccw projected
  arc A390 (11.9888, 101.293) -> (9.9376, 96.9922) centre (36.3113, 87.0532) ccw projected
  arc A391 (9.9376, 96.9922) -> (8.4129, 97.1364) centre (0, 0) ccw projected
  arc A392 (8.4129, 97.1364) -> (7.204, 101.7453) centre (-19.356, 92.3153) ccw projected
  arc A393 (7.204, 101.7453) -> (5.6049, 101.8459) centre (0, 0) ccw projected
  arc A394 (5.6049, 101.8459) -> (3.8278, 97.4248) centre (30.7735, 89.1614) ccw projected
  arc A395 (3.8278, 97.4248) -> (2.2971, 97.4729) centre (0, 0) ccw projected
  arc A396 (2.2971, 97.4729) -> (0.8011, 101.9969) centre (-25.1143, 90.9178) ccw projected
  arc A397 (0.8011, 101.9969) -> (-0.8011, 101.9969) centre (0, 0) ccw projected
  arc A398 (-0.8011, 101.9969) -> (-2.2971, 97.4729) centre (25.1143, 90.9178) ccw projected
  arc A399 (-2.2971, 97.4729) -> (-3.8278, 97.4248) centre (0, 0) ccw projected
  arc A400 (-3.8278, 97.4248) -> (-5.6049, 101.8459) centre (-30.7735, 89.1614) ccw projected
  arc A401 (-5.6049, 101.8459) -> (-7.204, 101.7453) centre (0, 0) ccw projected
  circle A402 centre (0, 0) radius 10
  circle A403 centre (0, 0) radius 30
  point P0 (21.2132, -21.2132)
  point P1 (-21.2132, 21.2132)
  point P2 (-69.4823, 68.3993)
  dimension "d49" = 135
  dimension "d50" = 45
  dimension "d51" = 20
  dimension "d52" = 60
  constraints: 8 end point, 2 centre point, 2 coincident, 2 equal length, 2 horizontal, 2 point on circle
  measures "d49" angle of L1 L0
  measures "d50" angle of L2 L3
  measures "d51" diameter of A402
  measures "d52" diameter of A403
extrude "Extrusion2" cut sketch "Sketch3" against normal up to surface (20 mm away) contours L2 A402 L0 | L0 A402 L2 | A403 L2 A1 A246 A245 A244 A243 A242 A241 A240 A239 A238 A237 A236 A235 A234 A233 A232 A231 A230 A229 A228 A227 A226 A225 A224 A223 A222 A221 A220 A219 A218 A217 A216 A215 A214 A213 A212 A211 A210 A209 A208 A207 A206 A205 A204 A203 A202 A201 A200 A199 A198 A197 A196 A195 A194 A193 A192 A191 A190 A189 A188 A187 A186 A185 A184 A183 A182 A181 A180 A179 A178 A177 A176 A175 A174 A173 A172 A171 A170 A169 A168 A167 A166 A165 A164 A163 A162 A161 A160 A159 A158 A157 A156 A155 A154 A153 A152 A151 A150 A149 A148 A147 A146 A145 A144 A143 A142 A141 A140 A139 A138 A137 A136 A135 A134 A133 A132 A131 A130 A129 A128 A127 A126 A125 A124 A123 A122 A121 A120 A119 A118 A117 A116 A115 A114 A113 A112 A111 A110 A109 A108 A107 A106 A105 A104 A103 A102 A101 A100 A99 A98 A97 A96 A95 A94 A93 A92 A91 A90 A89 A88 A87 A86 A85 A84 A83 A82 A81 A80 A79 A78 A77 A76 A75 A74 A73 A72 A71 A70 A69 A68 A67 A66 A65 A64 A63 A62 A61 A60 A59 A58 A57 A56 A55 A54 A53 A52 A51 A50 A49 A48 A0 L0